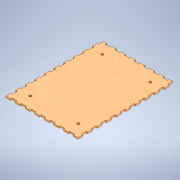
# Autodesk Inventor part: TableBottom
Saved by Autodesk Inventor 2021 (Build 250183000, 183)
## iProperties
Created: 2021-03-11
Part Number: TableBottom
Material: Wood (Cherry)
Document SubType Name: Modeling
Designer: ZiweZhang
Density: 0.63 g/cm^3
Appearance: Cherry - Natural Low Gloss
Author: ZiweZhang
Autodesk Inventor part; units mm, degrees
ref_plane "YZ Plane" through (0, 0, 0) normal (1, 0, 0) x (0, 1, 0)
ref_plane "XZ Plane" through (0, 0, 0) normal (0, 1, 0) x (-1, 0, 0)
ref_plane "XY Plane" through (0, 0, 0) normal (0, 0, 1) x (1, 0, 0)
sketch "Sketch2" plane through (0, 0, 0) normal (0, 1, 0) x (-1, 0, 0)
  line L0 (0, 0) -> (150, 0)
  line L1 (150, 0) -> (150, -200)
  line L2 (150, -200) -> (0, -200)
  line L3 (0, -200) -> (0, 0)
  point P0 (75, -100)
  dimension "d4" = 150
  dimension "d5" = 200
  constraints: 8 end point, 2 parallel, 1 horizontal, 1 perpendicular
  measures "d4" distance of L1.end L2.end
  measures "d5" distance of L0.end L1.end
extrude "Extrusion2" add sketch "Sketch2" along normal blind 3
sketch "Sketch3" plane through (0, 0, 0) normal (0, -1, 0) x (1, 0, 0)
  line L0 (-150, 0) -> (0, 0) projected
  line L1 (0, 0) -> (-10, 0)
  line L2 (-10, 0) -> (-10, -3)
  line L3 (-10, -3) -> (-20, -3)
  line L4 (-20, -3) -> (-20, 0)
  line L5 (-20, 0) -> (-30, 0)
  line L6 (-30, -3) -> (-40, -3)
  line L7 (-30, 0) -> (-30, -3)
  line L8 (-40, -3) -> (-40, 0)
  line L9 (-40, 0) -> (-50, 0)
  line L10 (-50, -3) -> (-60, -3)
  line L11 (-50, 0) -> (-50, -3)
  line L12 (-60, -3) -> (-60, 0)
  line L13 (-60, 0) -> (-70, 0)
  line L14 (-70, -3) -> (-80, -3)
  line L15 (-70, 0) -> (-70, -3)
  line L16 (-80, -3) -> (-80, 0)
  line L17 (-80, 0) -> (-90, 0)
  line L18 (-90, -3) -> (-100, -3)
  line L19 (-90, 0) -> (-90, -3)
  line L20 (-100, -3) -> (-100, 0)
  line L21 (-100, 0) -> (-110, 0)
  line L22 (-110, -3) -> (-120, -3)
  line L23 (-110, 0) -> (-110, -3)
  line L24 (-120, -3) -> (-120, 0)
  line L25 (-120, 0) -> (-130, 0)
  line L26 (-130, -3) -> (-140, -3)
  line L27 (-130, 0) -> (-130, -3)
  line L28 (-140, -3) -> (-140, 0)
  line L29 (-140, 0) -> (-150, 0)
  line L30 (-150, -200) -> (-150, 0) projected
  line L31 (-150, 0) -> (-150, -10)
  line L32 (-150, -10) -> (-147, -10)
  line L33 (-147, -10) -> (-147, -20)
  line L34 (-147, -20) -> (-150, -20)
  line L35 (-147, -30) -> (-147, -40)
  line L36 (-147, -40) -> (-150, -40)
  line L37 (-150, -30) -> (-147, -30)
  line L38 (-150, -20) -> (-150, -30)
  line L39 (-147, -50) -> (-147, -60)
  line L40 (-147, -60) -> (-150, -60)
  line L41 (-150, -50) -> (-147, -50)
  line L42 (-150, -40) -> (-150, -50)
  line L43 (-147, -70) -> (-147, -80)
  line L44 (-147, -80) -> (-150, -80)
  line L45 (-150, -70) -> (-147, -70)
  line L46 (-150, -60) -> (-150, -70)
  line L47 (-147, -90) -> (-147, -100)
  line L48 (-147, -100) -> (-150, -100)
  line L49 (-150, -90) -> (-147, -90)
  line L50 (-150, -80) -> (-150, -90)
  line L51 (-147, -110) -> (-147, -120)
  line L52 (-147, -120) -> (-150, -120)
  line L53 (-150, -110) -> (-147, -110)
  line L54 (-150, -100) -> (-150, -110)
  line L55 (-147, -130) -> (-147, -140)
  line L56 (-147, -140) -> (-150, -140)
  line L57 (-150, -130) -> (-147, -130)
  line L58 (-150, -120) -> (-150, -130)
  line L59 (-147, -150) -> (-147, -160)
  line L60 (-147, -160) -> (-150, -160)
  line L61 (-150, -150) -> (-147, -150)
  line L62 (-150, -140) -> (-150, -150)
  line L63 (-147, -170) -> (-147, -180)
  line L64 (-147, -180) -> (-150, -180)
  line L65 (-150, -170) -> (-147, -170)
  line L66 (-150, -160) -> (-150, -170)
  line L67 (-150, -180) -> (-150, -190)
  line L68 (-150, -190) -> (-147, -190)
  line L69 (0, 0) -> (0, -10)
  line L70 (0, 0) -> (0, -200) projected
  line L71 (-3, -10) -> (-3, -20)
  line L72 (-3, -20) -> (0, -20)
  line L73 (0, -20) -> (0, -30)
  line L74 (0, -30) -> (-3, -30)
  line L75 (-3, -30) -> (-3, -40)
  line L76 (-3, -40) -> (0, -40)
  line L77 (0, -40) -> (0, -50)
  line L78 (0, -50) -> (-3, -50)
  line L79 (-3, -50) -> (-3, -60)
  line L80 (-3, -60) -> (0, -60)
  line L81 (0, -60) -> (0, -70)
  line L82 (0, -70) -> (-3, -70)
  line L83 (-3, -70) -> (-3, -80)
  line L84 (-3, -80) -> (0, -80)
  line L85 (0, -80) -> (0, -90)
  line L86 (0, -90) -> (-3, -90)
  line L87 (-3, -90) -> (-3, -100)
  line L88 (-3, -100) -> (0, -100)
  line L89 (0, -100) -> (0, -110)
  line L90 (0, -110) -> (-3, -110)
  line L91 (-3, -110) -> (-3, -120)
  line L92 (-3, -120) -> (0, -120)
  line L93 (0, -120) -> (0, -130)
  line L94 (0, -130) -> (-3, -130)
  line L95 (-3, -130) -> (-3, -140)
  line L96 (-3, -140) -> (0, -140)
  line L97 (0, -140) -> (0, -150)
  line L98 (0, -150) -> (-3, -150)
  line L99 (-3, -150) -> (-3, -160)
  line L100 (-3, -160) -> (0, -160)
  line L101 (0, -160) -> (0, -170)
  line L102 (0, -170) -> (-3, -170)
  line L103 (-3, -170) -> (-3, -180)
  line L104 (-3, -180) -> (0, -180)
  line L105 (0, -180) -> (0, -190)
  line L106 (0, -190) -> (-3, -190)
  line L107 (-3, -190) -> (-3, -200)
  line L108 (0, -200) -> (-150, -200) projected
  line L109 (-147, -190) -> (-147, -200)
  line L110 (0, -10) -> (-3, -10)
  line L111 (-147, -200) -> (-140, -200)
  line L112 (-140, -197) -> (-130, -197)
  line L113 (-130, -197) -> (-130, -200)
  line L114 (-120, -200) -> (-120, -197)
  line L115 (-120, -197) -> (-110, -197)
  line L116 (-110, -197) -> (-110, -200)
  line L117 (-100, -200) -> (-100, -197)
  line L118 (-100, -197) -> (-90, -197)
  line L119 (-90, -197) -> (-90, -200)
  line L120 (-80, -200) -> (-80, -197)
  line L121 (-80, -197) -> (-70, -197)
  line L122 (-70, -197) -> (-70, -200)
  line L123 (-60, -200) -> (-60, -197)
  line L124 (-60, -197) -> (-50, -197)
  line L125 (-50, -197) -> (-50, -200)
  line L126 (-40, -200) -> (-40, -197)
  line L127 (-40, -197) -> (-30, -197)
  line L128 (-30, -197) -> (-30, -200)
  line L129 (-20, -200) -> (-20, -197)
  line L130 (-20, -197) -> (-10, -197)
  line L131 (-10, -197) -> (-10, -200)
  line L132 (-140, -197) -> (-140, -200)
  dimension "d8" = 10
  dimension "d9" = 3
  dimension "d10" = 10
  dimension "d13" = 20
  dimension "d18" = 10
  dimension "d19" = 3
  dimension "d20" = 10
  dimension "d23" = 20
  dimension "d28" = 10
  constraints: 258 end point, 50 point on line, 40 vertical alignment, 25 perpendicular, 18 parallel, 17 collinear, 13 vertical, 4 horizontal, 77 other
  measures "d8" distance of L0.end L1.end
  measures "d9" distance of L1.end L2.end
  measures "d10" distance of L2.end L3.end
  measures "d13" distance of L0.end L5.start
  measures "d18" distance of L0.start L31.end
  measures "d19" distance of L31.end L32.end
  measures "d20" distance of L32.end L33.end
  measures "d23" distance of L32.end L35.start
  measures "d28" distance of L64.end L67.end
extrude "Extrusion3" cut sketch "Sketch3" against normal blind 3 contours L0 L28 L26 L27 L24 L22 L23 L20 L18 L19 L16 L14 L15 L12 L10 L11 L8 L6 L7 L4 L3 L2 L69 L110 L71 L72 L70 L74 L75 L76 L78 L79 L80 L82 L83 L84 L86 L87 L88 L90 L91 L92 L94 L95 L96 L98 L99 L100 L102 L103 L104 L106 L107 L108 L131 L130 L129 L128 L127 L126 L125 L124 L123 L122 L121 L120 L119 L118 L117 L116 L115 L114 L113 L112 L132 L109 L68 L30 L64 L63 L65 L60 L59 L61 L56 L55 L57 L52 L51 L53 L48 L47 L49 L44 L43 L45 L40 L39 L41 L36 L35 L37 L34 L33 L32 keep common part
sketch "Sketch5" plane through (0, 3, 0) normal (0, 1, 0) x (1, 0, 0)
  line L0 (-150, 10) -> (-150, 0) projected
  circle A0 centre (-24.8562, 25.4431) radius 2.5
  circle A1 centre (-124.8562, 25.4431) radius 2.5
  circle A2 centre (-24.8562, 175.4431) radius 2.5
  circle A3 centre (-124.8562, 175.4431) radius 2.5
  point P0 (0, 0)
  point P1 (0, 0)
  point P2 (-75, 100)
  dimension "d38" = 5
  dimension "d39" = 100
  dimension "d40" = 150
  constraints: 4 centre point
  measures "d38" diameter of A0
  measures "d39" distance of A0.centre A1.centre
  measures "d40" distance of A0.centre A2.centre
extrude "Extrusion4" cut sketch "Sketch5" against normal blind 2
body "Solid2"
